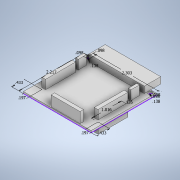
# Autodesk Inventor part: MSP432CoreModule
Saved by Autodesk Inventor 2022.2 (Build 262287000, 287)
## iProperties
Created: 2022-01-14
Part Number: MSP432CoreModule
Material: Generic
Document SubType Name: Modeling
Designer: Max
Density: 1 g/cm^3
Appearance: Default
Author: Max
Autodesk Inventor part; units mm, degrees
ref_plane "YZ Plane" through (0, 0, 0) normal (1, 0, 0) x (0, 1, 0)
ref_plane "XZ Plane" through (0, 0, 0) normal (0, 1, 0) x (-1, 0, 0)
ref_plane "XY Plane" through (0, 0, 0) normal (0, 0, 1) x (1, 0, 0)
sketch "Base Board" plane through (0, 0, 0) normal (0, 1, 0) x (-1, 0, 0)
  line L0 (-28.8413, 27.4927) -> (29.6587, 27.4927)
  line L1 (29.6587, 27.4927) -> (29.6587, -28.8073)
  line L2 (29.6587, -28.8073) -> (-28.8413, -28.8073)
  line L3 (-28.8413, -28.8073) -> (-28.8413, 27.4927)
  circle A0 centre (27.1587, -26.3073) radius 1.755
  circle A1 centre (-26.3413, -26.3073) radius 1.755
  line L4 (-23.8413, 16.4927) -> (-20.6413, 16.4927)
  line L5 (-20.6413, 16.4927) -> (-20.6413, -9.3073)
  line L6 (-20.6413, -9.3073) -> (-23.8413, -9.3073)
  line L7 (-23.8413, -9.3073) -> (-23.8413, 16.4927)
  line L8 (24.6587, 16.4927) -> (21.4587, 16.4927)
  line L9 (21.4587, 16.4927) -> (21.4587, -9.3073)
  line L10 (21.4587, -9.3073) -> (24.6587, -9.3073)
  line L11 (24.6587, -9.3073) -> (24.6587, 16.4927)
  point P0 (0, 0)
  dimension "d0" = 58.5
  dimension "d1" = 56.3
  dimension "d2" = 3.51
  dimension "d3" = 2.5
  dimension "d4" = 2.5
  dimension "d5" = 3.51
  dimension "d6" = 2.5
  dimension "d7" = 2.5
  dimension "d19" = 3.2
  dimension "d20" = 25.8
  dimension "d23" = 11
  dimension "d24" = 5
  dimension "d25" = 11
  dimension "d26" = 5
  constraints: 24 end point, 4 parallel, 2 centre point, 2 horizontal, 2 perpendicular
  measures "d0" distance of L1.end L2.end
  measures "d1" distance of L0.end L1.end
  measures "d2" diameter of A0
  measures "d3" distance from line of L1 A0.centre
  measures "d4" distance from line of L2 A0.centre
  measures "d5" diameter of A1
  measures "d6" distance from line of L3 A1.centre
  measures "d7" distance from line of L2 A1.centre
  measures "d19" distance of L5.end L6.end
  measures "d20" distance of L4.end L5.end
  measures "d23" distance between parallel lines of L0 L4
  measures "d24" distance between parallel lines of L3 L7
  measures "d25" distance between parallel lines of L0 L8
  measures "d26" distance between parallel lines of L1 L11
extrude "Base Board Extrusion" add sketch "Base Board" along normal blind 1.5 contours L0 L1 L2 L3 | L4 L5 L6 L7 | L11 L10 L9 L8
sketch "Sketch2" plane through (0, 1.5, 0) normal (0, 1, 0) x (1, 0, 0)
  line L0 (-23.9587, 28.2917) -> (24.0413, 28.2917)
  line L1 (24.0413, 28.2917) -> (24.0413, 23.2917)
  line L2 (24.0413, 23.2917) -> (-23.9587, 23.2917)
  line L3 (-23.9587, 23.2917) -> (-23.9587, 28.2917)
  line L4 (-29.6587, 28.8073) -> (-29.6587, -27.4927) projected
  point P0 (0, 0)
  dimension "d10" = 48
  dimension "d11" = 5
  dimension "d12" = 5.7
  constraints: 8 end point, 2 parallel, 1 horizontal, 1 perpendicular
  measures "d10" distance of L1.end L2.end
  measures "d11" distance of L0.end L1.end
  measures "d12" distance between parallel lines of L4 L3
extrude "RightAngleconnectorsBase" add sketch "Sketch2" along normal blind 5.5
sketch "Sketch4" plane through (24.0413, 1.5, -28.2917) normal (0, 0, -1) x (-1, 0, 0)
  line L0 (48, 5.5) -> (0, 5.5) projected
  line L1 (48, 0) -> (48, 5.5) projected
  line L2 (0, 5.5) -> (48, 5.5)
  line L3 (48, 5.5) -> (48, 0)
  line L4 (48, 0) -> (0, 0)
  line L5 (0, 0) -> (0, 5.5)
  point P0 (24.0413, -1.5)
  constraints: 8 end point, 2 parallel, 1 horizontal, 1 perpendicular
extrude "RightAnglePins" add sketch "Sketch4" along normal blind 9.2
extrude "Main IO" add sketch "Base Board" along normal mid plane 18.5 contours L4 L5 L6 L7 | L11 L10 L9 L8
sketch "Sketch6" plane through (0, 1.5, 0) normal (0, 1, 0) x (1, 0, 0)
  line L0 (18.8413, -26.9927) -> (-6.1587, -26.9927)
  line L1 (-6.1587, -26.9927) -> (-6.1587, -23.9927)
  line L2 (-6.1587, -23.9927) -> (18.8413, -23.9927)
  line L3 (18.8413, -23.9927) -> (18.8413, -26.9927)
  line L4 (28.8413, -27.4927) -> (28.8413, 28.8073) projected
  line L5 (-29.6587, -27.4927) -> (28.8413, -27.4927) projected
  point P0 (0, 0)
  dimension "d29" = 25
  dimension "d30" = 3
  dimension "d31" = 10
  dimension "d32" = 0.5
  constraints: 8 end point, 2 parallel, 1 horizontal, 1 perpendicular
  measures "d29" distance of L1.end L2.end
  measures "d30" distance of L0.end L1.end
  measures "d31" distance between parallel lines of L4 L3
  measures "d32" distance between parallel lines of L5 L0
extrude "Emulator Pins" add sketch "Sketch6" along normal blind 9
sketch "Sketch7" plane through (0, 1.5, 0) normal (0, 1, 0) x (1, 0, 0)
  line L0 (23.5413, 12.3073) -> (21.2413, 12.3073)
  line L1 (21.2413, 12.3073) -> (21.2413, 19.5573)
  line L2 (21.2413, 19.5573) -> (23.5413, 19.5573)
  line L3 (23.5413, 19.5573) -> (23.5413, 12.3073)
  line L4 (28.8413, -27.4927) -> (28.8413, 28.8073) projected
  line L5 (23.8413, 9.3073) -> (20.6413, 9.3073) projected
  line L6 (-29.6587, -27.4927) -> (28.8413, -27.4927) projected
  line L7 (-24.3587, 12.3073) -> (-22.0587, 12.3073)
  line L8 (-22.0587, 12.3073) -> (-22.0587, 19.5573)
  line L9 (-22.0587, 19.5573) -> (-24.3587, 19.5573)
  line L10 (-24.3587, 19.5573) -> (-24.3587, 12.3073)
  point P0 (0, 0)
  dimension "d35" = 2.3
  dimension "d36" = 7.25
  dimension "d37" = 5.3
  dimension "d38" = 3
  constraints: 16 end point, 2 parallel, 1 horizontal, 1 perpendicular
  measures "d35" distance of L1.end L2.end
  measures "d36" distance of L0.end L1.end
  measures "d37" distance between parallel lines of L4 L3
  measures "d38" distance between parallel lines of L5 L0
extrude "Power Pins" add sketch "Sketch7" along normal blind 8
body "Solid1"
